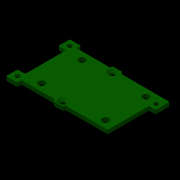
# Autodesk Inventor part: hw_DAA - PCB Sensor
Saved by Autodesk Inventor 2018 (Build 220112000, 112)
## iProperties
Created: 2024-03-13
Part Number: hw_DAA - PCB Sensor
Material: PCB
Document SubType Name: Modeling
Designer: cda1
Density: 4 g/cm^3
Appearance: PCB
Author: cda1
Autodesk Inventor part; units mm, degrees
ref_plane "YZ Plane" through (0, 0, 0) normal (1, 0, 0) x (0, 1, 0)
ref_plane "XZ Plane" through (0, 0, 0) normal (0, 1, 0) x (-1, 0, 0)
ref_plane "XY Plane" through (0, 0, 0) normal (0, 0, 1) x (1, 0, 0)
sketch "Boceto1" plane through (0, 0, 0) normal (0, 0, 1) x (1, 0, 0)
  line L0 (-26, 17) -> (26, 17)
  line L1 (26, 17) -> (26, -17)
  line L2 (26, -17) -> (-26, -17)
  line L3 (-26, -17) -> (-26, 17)
  line L4 (-26, 17) -> (26, -17) construction
  line L5 (26, 17) -> (-26, -17) construction
  point P0 (0, 0)
  dimension "d0" = 52
  dimension "d1" = 34
  constraints: 12 end point, 2 midpoint, 2 parallel, 1 horizontal, 1 perpendicular
  measures "d0" distance of L1.end L2.end
  measures "d1" distance of L0.end L1.end
extrude "Extrusión1" add sketch "Boceto1" against normal blind 1.742
fillet "Empalme1" radius 0.5 4 edges at (26, 17, -0.871) (-26, 17, -0.871) (-26, -17, -0.871) (26, -17, -0.871)
sketch "Boceto2" plane through (0, 0, -1.742) normal (0, 0, -1) x (-1, 0, 0)
  line L0 (-25.5, -17) -> (25.5, -17) projected
  line L1 (-25.5, -17) -> (25.5, -17) projected
  line L2 (22.8, -17) -> (26, -17)
  line L3 (26, -17) -> (26, 13)
  line L4 (26, 13) -> (22.8, 13)
  line L5 (22.8, 13) -> (22.8, -17)
  line L6 (26, 16.5) -> (26, -16.5) projected
  point P0 (0, 0)
  dimension "d5" = 3.2
  dimension "d6" = 30
  constraints: 8 end point, 2 parallel, 2 point on line, 1 horizontal, 1 perpendicular
  measures "d5" distance of L4.end L3.end
  measures "d6" distance of L3.end L2.end
extrude "Extrusión2" cut sketch "Boceto2" against normal through all
sketch "Boceto3" plane through (0, 0, -1.742) normal (0, 0, -1) x (-1, 0, 0)
  line L0 (22.8, 13) -> (26, 13) construction
  line L1 (26, 13) -> (26, 16.5) construction
  arc A0 (26, 16.5) -> (25.5, 17) centre (25.5, 16.5) ccw construction
  line L2 (25.5, 17) -> (-25.5, 17) construction
  arc A1 (-25.5, 17) -> (-26, 16.5) centre (-25.5, 16.5) ccw projected
  line L3 (-26, 16.5) -> (-26, -16.5) projected
  arc A2 (-26, -16.5) -> (-25.5, -17) centre (-25.5, -16.5) ccw projected
  line L4 (-25.5, -17) -> (22.8, -17) construction
  line L5 (22.8, -17) -> (22.8, 13) construction
  line L6 (25.5, 17) -> (-25.5, 17) projected
  line L7 (-25.5, 17) -> (-33.8, 17)
  line L8 (-33.8, 17) -> (-33.8, -17)
  arc A3 (-26, -16.5) -> (-25.5, -17) centre (-25.5, -16.5) ccw projected
  line L9 (-25.5, -17) -> (-33.8, -17)
  point P0 (0, 0)
  dimension "d10" = 8.3
  constraints: 6 end point, 1 collinear, 1 horizontal, 1 perpendicular
  measures "d10" distance of L2.end L7.end
extrude "Extrusión3" add sketch "Boceto3" against normal up to surface (1.742 mm away)
fillet "Empalme2" radius 3.5 2 edges at (33.8, -17, -0.871) (33.8, 17, -0.871)
fillet "Empalme3" radius 1 1 edges at (-22.8, -17, -0.871)
sketch "Boceto4" plane through (0, 0, -1.742) normal (0, 0, -1) x (-1, 0, 0)
  line L0 (-33.8, 13.5) -> (-33.8, -13.5) projected
  line L1 (-30.3, -17) -> (21.8, -17) projected
  line L2 (25.5, 17) -> (-30.3, 17) projected
  line L3 (26, 13) -> (26, 16.5) projected
  point P0 (0, 0)
  point P1 (-24.195, -13.82)
  point P2 (-30.62, 8.694)
  point P3 (18.5, 13.82)
  dimension "d15" = 9.605
  dimension "d16" = 3.18
  dimension "d17" = 8.306
  dimension "d18" = 3.18
  dimension "d19" = 7.5
  dimension "d20" = 3.18
  measures "d15" distance from line of L0 point (-24.195, -13.82)
  measures "d16" distance from line of L1 point (-24.195, -13.82)
  measures "d17" distance from line of L2 point (-30.62, 8.694)
  measures "d18" distance from line of L0 point (-30.62, 8.694)
  measures "d19" distance from line of L3 point (18.5, 13.82)
  measures "d20" distance from line of L2 point (18.5, 13.82)
hole "Agujero1" [suppressed]
sketch "Boceto11" plane through (0, 0, -1.742) normal (0, 0, -1) x (-1, 0, 0)
  line L0 (25.5, 17) -> (-30.3, 17) projected
  line L1 (16.4, 13.533) -> (16.4, -13.067)
  line L2 (-30.3, -17) -> (21.8, -17) projected
  line L3 (22.8, -16) -> (22.8, 13) projected
  line L4 (-33.8, 13.5) -> (-33.8, -13.5) projected
  line L5 (-32.8, 13.533) -> (16.4, 13.533)
  line L6 (-32.8, 13.533) -> (-32.8, -13.067)
  line L7 (-32.8, -13.067) -> (16.4, -13.067)
  line L8 (6.1, -14.067) -> (11.1, -14.067)
  line L9 (11.1, -14.067) -> (11.1, -13.067)
  line L10 (6.1, -14.067) -> (6.1, -13.067)
  line L11 (14.6, 13.533) -> (14.6, 14.533)
  line L12 (14.6, 14.533) -> (9.6, 14.533)
  line L13 (9.6, 14.533) -> (9.6, 13.533)
  line L14 (-32.8, 11.333) -> (-33.8, 11.333)
  line L15 (-32.8, 6.333) -> (-33.8, 6.333)
  line L16 (-33.8, 6.333) -> (-33.8, 11.333)
  arc A0 (-30.3, 17) -> (-33.8, 13.5) centre (-30.3, 13.5) ccw projected
  arc A1 (-33.8, -13.5) -> (-30.3, -17) centre (-30.3, -13.5) ccw projected
  arc A2 (21.8, -17) -> (22.8, -16) centre (21.8, -16) ccw projected
  line L17 (22.8, 13) -> (26, 13) projected
  line L18 (26, 13) -> (26, 16.5) projected
  arc A3 (26, 16.5) -> (25.5, 17) centre (25.5, 16.5) ccw projected
  point P0 (0, 0)
  dimension "d75" = 6.4
  dimension "d76" = 3.467
  dimension "d77" = 1
  dimension "d78" = 3.933
  dimension "d79" = 2.933
  dimension "d80" = 5
  dimension "d81" = 5.3
  dimension "d82" = 5
  dimension "d83" = 1.8
  dimension "d84" = 1
  dimension "d85" = 5
  dimension "d86" = 2.2
  constraints: 26 end point, 9 perpendicular, 8 point on line, 3 vertical, 1 horizontal
  measures "d75" distance between parallel lines of L3 L1
  measures "d76" distance between parallel lines of L0 L5
  measures "d77" distance between parallel lines of L4 L6
  measures "d78" distance between parallel lines of L2 L7
  measures "d79" distance between parallel lines of L2 L8
  measures "d80" distance of L8.start L8.end
  measures "d81" distance from line of L1 L8.end
  measures "d82" distance of L11.end L12.end
  measures "d83" distance between parallel lines of L1 L11
  measures "d84" distance between parallel lines of L5 L12
  measures "d85" distance between parallel lines of L14 L15
  measures "d86" distance between parallel lines of L5 L14
extrude "Extrusión8" cut sketch "Boceto11" against normal through all contours A3 L18 L17 L3 A2 L2 A1 L4 L15 L6 L7 L10 L8 L9 L1 L5 L11 L12 L13 L14 A0 L0
fillet "Empalme5" radius 0.5 16 edges at (32.8, 13.533, -0.871) (32.8, 11.333, -0.871) (33.8, 11.333, -0.871) (33.8, 6.333, -0.871) (32.8, 6.333, -0.871) (32.8, -13.067, -0.871) (-6.1, -13.067, -0.871) (-6.1, -14.067, -0.871) (-11.1, -14.067, -0.871) (-11.1, -13.067, -0.871) (-16.4, -13.067, -0.871) (-16.4, 13.533, -0.871) (-14.6, 13.533, -0.871) (-14.6, 14.533, -0.871) (-9.6, 14.533, -0.871) (-9.6, 13.533, -0.871)
sketch "Boceto13" plane through (0, 0, -1.742) normal (0, 0, -1) x (-1, 0, 0)
  line L0 (9.1, 13.533) -> (-32.3, 13.533) projected
  line L1 (-32.8, 13.033) -> (-32.8, 11.833) projected
  line L2 (-32.3, -13.067) -> (5.6, -13.067) projected
  line L3 (-32.8, 5.833) -> (-32.8, -12.567) projected
  line L4 (16.4, -12.567) -> (16.4, 13.033) projected
  point P0 (0, 0)
  point P1 (3.9, 9.233)
  point P2 (3.9, -8.767)
  point P3 (-24.5, 9.233)
  point P4 (-24.5, -8.767)
  dimension "d103" = 4.3
  dimension "d105" = 4.3
  dimension "d137" = 12.5
  dimension "d188" = 28.4
  constraints: 2 horizontal alignment, 2 vertical alignment
  measures "d103" distance from line of L0 point (3.9, 9.233)
  measures "d105" distance from line of L2 point (3.9, -8.767)
  measures "d137" distance from line of L4 point (3.9, -8.767)
  measures "d188" distance of point (3.9, 9.233) point (-24.5, 9.233)
hole "Agujero5" at (-3.9, 9.233, -1.742) at (-3.9, -8.767, -1.742) at (24.5, 9.233, -1.742) at (24.5, -8.767, -1.742) direction (0, 0, 1) diameter 3 end through all
sketch "Boceto15" plane through (0, 0, 0) normal (0, 0, 1) x (1, 0, 0)
  line L0 (-16.4, 13.033) -> (-16.4, -12.567) projected
  line L1 (32.3, 13.533) -> (-9.1, 13.533) projected
  line L2 (-5.6, -13.067) -> (32.3, -13.067) projected
  point P0 (0, 0)
  point P1 (7.65, 11.233)
  point P2 (7.65, -10.767)
  dimension "d126" = 24.05
  dimension "d127" = 2.3
  dimension "d128" = 2.3
  constraints: 1 vertical alignment
  measures "d126" distance from line of L0 point (7.65, -10.767)
  measures "d127" distance from line of L1 point (7.65, 11.233)
  measures "d128" distance from line of L2 point (7.65, -10.767)
hole "Agujero7" at (7.65, 11.233, 0) at (7.65, -10.767, 0) direction (0, 0, -1) diameter 2 end through all countersink diameter 4 countersink angle 90
sketch "Boceto16" plane through (0, 0, -1.742) normal (0, 0, -1) x (-1, 0, 0)
  circle A0 centre (-24.5, 9.233) radius 1.5 projected
  circle A1 centre (3.9, 9.233) radius 1.5 projected
  circle A2 centre (3.9, -8.767) radius 1.5 projected
  circle A3 centre (3.9, -8.767) radius 2.65
  circle A4 centre (3.9, 9.233) radius 2.65
  circle A5 centre (-24.5, 9.233) radius 2.65
  circle A6 centre (-24.5, -8.767) radius 1.5 projected
  circle A7 centre (-24.5, -8.767) radius 2.65
  point P0 (0, 0)
  dimension "d138" = 5.3
  dimension "d139" = 5.3
  dimension "d140" = 5.3
  dimension "d183" = 5.3
  constraints: 4 centre point, 4 coincident
  measures "d138" diameter of A3
  measures "d139" diameter of A4
  measures "d140" diameter of A5
  measures "d183" diameter of A7
extrude "Extrusión9" add sketch "Boceto16" along normal blind 0.0001
sketch "Boceto18" plane through (0, 0, -1.742) normal (0, 0, -1) x (-1, 0, 0)
  line L0 (12.1724, -6.0157) -> (12.1724, 6.9843) projected
  line L1 (12.1724, 6.9843) -> (13.1724, 6.9843) construction
  line L2 (13.1724, 6.9843) -> (15.6724, 6.9843) construction
  line L3 (13.1724, -6.0157) -> (12.1724, -6.0157) construction
  line L4 (15.6724, -6.0157) -> (13.1724, -6.0157) construction
  line L5 (12.1724, 6.9843) -> (12.1724, 7.9843)
  line L6 (12.1724, 7.9843) -> (16.4, 7.9843)
  line L7 (12.1724, -6.0157) -> (12.1724, -7.0157)
  line L8 (12.1724, -7.0157) -> (16.4, -7.0157)
  line L9 (16.4, -12.567) -> (16.4, 13.033) projected
  line L10 (16.4, -7.0157) -> (16.4, 7.9843)
  point P0 (0, 0)
  dimension "d145" = 1
  dimension "d146" = 1
  constraints: 10 end point, 2 perpendicular, 2 vertical, 1 collinear, 1 point on line
  measures "d145" distance of L0.end L5.end
  measures "d146" distance of L0.start L7.end
extrude "Extrusión11" cut sketch "Boceto18" against normal up to surface (1.742 mm away)
fillet "Empalme6" radius 0.5 2 edges at (-16.4, 7.9843, -0.871) (-16.4, -7.0157, -0.871)
sketch "Boceto19" plane through (0, 0, 0) normal (0, 0, 1) x (1, 0, 0)
  line L0 (-16.4, 13.533) -> (-14.6, 13.533)
  line L1 (-14.6, 13.533) -> (-14.6, -13.067)
  line L2 (-14.6, -13.067) -> (-16.4, -13.067)
  line L3 (-16.4, -13.067) -> (-16.4, 13.533)
  line L4 (-16.4, 8.4843) -> (-16.4, 13.033) projected
  line L5 (-16.4, 9.333) -> (-11.2, 9.333)
  line L6 (-11.2, 9.333) -> (-11.2, -8.867)
  line L7 (-11.2, -8.867) -> (-16.4, -8.867)
  line L8 (-16.4, -8.867) -> (-16.4, 9.333)
  line L9 (-9.6, 13.533) -> (5.4, 13.533)
  line L10 (5.4, 13.533) -> (5.4, 12.533)
  line L11 (5.4, 12.533) -> (-9.6, 12.533)
  line L12 (-9.6, 12.533) -> (-9.6, 13.533)
  line L13 (9.9, 13.533) -> (32.8, 13.533)
  line L14 (32.8, 13.533) -> (32.8, 12.533)
  line L15 (32.8, 12.533) -> (9.9, 12.533)
  line L16 (9.9, 12.533) -> (9.9, 13.533)
  line L17 (32.8, 6.333) -> (31.8, 6.333)
  line L18 (31.8, 6.333) -> (31.8, -13.067)
  line L19 (31.8, -13.067) -> (32.8, -13.067)
  line L20 (32.8, -13.067) -> (32.8, 6.333)
  line L21 (9.9, -12.067) -> (32.8, -12.067)
  line L22 (32.8, -12.067) -> (32.8, -13.067)
  line L23 (32.8, -13.067) -> (9.9, -13.067)
  line L24 (9.9, -13.067) -> (9.9, -12.067)
  line L25 (5.4, -12.067) -> (-9.6, -12.067)
  line L26 (-9.6, -12.067) -> (-9.6, -14.067)
  line L27 (-9.6, -14.067) -> (5.4, -14.067)
  line L28 (5.4, -14.067) -> (5.4, -12.067)
  line L29 (31.8, 13.533) -> (33.8, 13.533)
  line L30 (33.8, 13.533) -> (33.8, 11.333)
  line L31 (33.8, 11.333) -> (31.8, 11.333)
  line L32 (31.8, 11.333) -> (31.8, 13.533)
  line L33 (33.8, 11.333) -> (33.7, 11.333)
  line L34 (33.7, 11.333) -> (33.7, 5.833)
  line L35 (33.7, 5.833) -> (33.8, 5.833)
  line L36 (33.8, 5.833) -> (33.8, 11.333)
  line L37 (33.8, 5.833) -> (32.8, 5.833)
  line L38 (32.8, 5.833) -> (32.8, 6.333)
  line L39 (32.8, 6.333) -> (33.8, 6.333)
  line L40 (33.8, 6.333) -> (33.8, 5.833)
  line L41 (-14.6, 13.533) -> (-16.4, 13.533)
  line L42 (-16.4, 13.533) -> (-16.4, 14.533)
  line L43 (-16.4, 14.533) -> (-14.6, 14.533)
  line L44 (-14.6, 14.533) -> (-14.6, 13.533)
  line L45 (-14.6, 14.533) -> (-9.1, 14.533)
  line L46 (-9.1, 14.533) -> (-9.1, 14.433)
  line L47 (-9.1, 14.433) -> (-14.6, 14.433)
  line L48 (-14.6, 14.433) -> (-14.6, 14.533)
  line L49 (-9.1, 14.533) -> (-9.6, 14.533)
  line L50 (-9.6, 14.533) -> (-9.6, 13.533)
  line L51 (-9.6, 13.533) -> (-9.1, 13.533)
  line L52 (-9.1, 13.533) -> (-9.1, 14.533)
  line L53 (-9.6, -14.067) -> (-11.1, -14.067)
  line L54 (-11.1, -14.067) -> (-11.1, -13.967)
  line L55 (-11.1, -13.967) -> (-9.6, -13.967)
  line L56 (-9.6, -13.967) -> (-9.6, -14.067)
  point P0 (0, 0)
  point P1 (-15.9, 13.533)
  point P2 (-15.9, -13.067)
  point P3 (-11.2, 0.233)
  point P4 (-16.4, 0.233)
  point P5 (32.3, 13.533)
  point P6 (32.8, 13.033)
  point P7 (32.3, -13.067)
  point P8 (32.8, -12.567)
  point P9 (-6.6, -14.067)
  point P10 (32.8, 13.033)
  point P11 (33.75, 5.833)
  point P12 (-14.1, 14.533)
  point P13 (-11.1, -14.017)
  point P14 (-11.1, -13.567)
  dimension "d150" = 1.8
  dimension "d151" = 18.2
  dimension "d152" = 5.2
  dimension "d153" = 1
  dimension "d154" = 15
  dimension "d155" = 0.5
  dimension "d156" = 1
  dimension "d157" = 22.9
  dimension "d158" = 1
  dimension "d159" = 19.4
  dimension "d160" = 1
  dimension "d161" = 2
  dimension "d162" = 22.9
  dimension "d163" = 15
  dimension "d164" = 4.5
  dimension "d165" = 2.2
  dimension "d166" = 2
  dimension "d167" = 1
  dimension "d168" = 0.1
  dimension "d169" = 0.1
  dimension "d170" = 0.1
  constraints: 112 end point, 28 parallel, 14 horizontal, 14 perpendicular, 11 point on line, 8 midpoint, 2 horizontal alignment, 1 vertical alignment
  measures "d150" distance of L0.start L0.end
  measures "d151" distance between parallel lines of L7 L5
  measures "d152" distance of L5.start L5.end
  measures "d153" distance of L9.end L10.end
  measures "d154" distance between parallel lines of L10 L12
  measures "d155" distance from line of L51.end L12
  measures "d156" distance of L15.end L13.start
  measures "d157" distance of L13.start L13.end
  measures "d158" distance of L18.end L19.end
  measures "d159" distance of L19.end L17.start
  measures "d160" distance of L21.end L22.end
  measures "d161" distance of L26.end L25.end
  measures "d162" distance between parallel lines of L22 L24
  measures "d163" distance of L26.end L27.end
  measures "d164" distance between parallel lines of L28 L24
  measures "d165" distance of L29.end L30.end
  measures "d166" distance between parallel lines of L30 L32
  measures "d167" distance from line of L30 point (32.8, 13.033)
  measures "d168" distance of L34.end L35.end
  measures "d169" distance of L45.end L46.end
  measures "d170" distance of L53.end L54.end
extrude "Extrusión12" cut sketch "Boceto19" against normal through all
sketch "Boceto20" plane through (0, 0, -1.742) normal (0, 0, -1) x (-1, 0, 0)
  line L0 (14.6, -13.067) -> (11.6, -13.067) projected
  line L1 (9.6, -13.967) -> (14.6, -13.967)
  line L2 (14.6, -13.967) -> (14.6, -13.067)
  line L3 (14.6, -13.067) -> (9.6, -13.067)
  line L4 (9.6, -13.067) -> (9.6, -13.967)
  point P0 (0, 0)
  constraints: 8 end point, 2 parallel, 1 horizontal, 1 perpendicular
extrude "Extrusión13" add sketch "Boceto20" against normal up to surface (1.742 mm away)
sketch "Boceto12" plane through (0, 0, -1.742) normal (0, 0, -1) x (-1, 0, 0)
  line L0 (-33.8, 10.833) -> (-33.8, 6.833) construction
  line L1 (9.1, 13.533) -> (-32.3, 13.533) construction
  line L2 (16.4, -12.567) -> (16.4, 13.033) construction
  line L3 (14.1, 14.533) -> (10.1, 14.533) construction
  line L4 (6.6, -14.067) -> (10.6, -14.067) construction
  point P0 (0, 0)
  point P1 (-29.521, 8.811)
  point P2 (12.1, 11.889)
  point P3 (12.1, -11.387)
  dimension "d90" = 4.279
  dimension "d91" = 4.722
  dimension "d92" = 4.3
  dimension "d93" = 2.644
  dimension "d94" = 4.3
  dimension "d95" = 2.68
  measures "d90" distance from line of L0 point (-29.521, 8.811)
  measures "d91" distance from line of L1 point (-29.521, 8.811)
  measures "d92" distance from line of L2 point (12.1, 11.889)
  measures "d93" distance from line of L3 point (12.1, 11.889)
  measures "d94" distance from line of L2 point (12.1, -11.387)
  measures "d95" distance from line of L4 point (12.1, -11.387)
hole "Agujero4" at (29.521, 8.811, -1.742) at (-12.1, 11.889, -1.742) at (-12.1, -11.387, -1.742) direction (0, 0, 1) diameter 2 end through all countersink diameter 4 countersink angle 90
fillet "Empalme7" radius 0.5 24 edges at (31.8, 12.533, -0.871) (31.8, 11.333, -0.871) (33.7, 11.1331, -0.871) (33.7, 6.5329, -0.871) (31.8, 6.333, -0.871) (31.8, -12.067, -0.871) (9.9, -12.067, -0.871) (9.9, -13.067, -0.871) (5.4, -12.067, -0.871) (5.4, -13.067, -0.871) (-9.6, -12.067, -0.871) (-9.6, -13.967, -0.871) (-14.6, -13.967, -0.871) (-14.6, -8.867, -0.871) (-11.2, -8.867, -0.871) (-11.2, 9.333, -0.871) (-14.6, 9.333, -0.871) (-14.4001, 14.433, -0.871) (-9.7999, 14.433, -0.871) (-9.6, 12.533, -0.871) (5.4, 13.533, -0.871) (5.4, 12.533, -0.871) (9.9, 13.533, -0.871) (9.9, 12.533, -0.871)
sketch "Boceto21" plane through (0, 0, -1.742) normal (0, 0, -1) x (-1, 0, 0)
  line L0 (-33.2, 6.333) -> (-32.3, 6.333) construction
  arc A0 (-31.8, 5.833) -> (-32.3, 6.333) centre (-32.3, 5.833) ccw construction
  line L1 (-31.8, 5.833) -> (-31.8, -11.567) construction
  line L2 (-31.3, -12.067) -> (-10.4, -12.067) construction
  line L3 (-32.3, 6.333) -> (-33.2, 6.333) projected
  line L4 (-33.2, 6.333) -> (-30.8, 6.333)
  line L5 (-30.8, 6.333) -> (-30.8, -12.067)
  line L6 (-30.8, -12.067) -> (-33.2, -12.067)
  line L7 (-33.2, -12.067) -> (-33.2, 6.333)
  point P0 (0, 0)
  dimension "d176" = 1
  constraints: 8 end point, 2 parallel, 1 horizontal, 1 perpendicular, 1 point on line
  measures "d176" distance between parallel lines of L1 L5
extrude "Extrusión14" cut sketch "Boceto21" against normal up to surface (1.742 mm away)
fillet "Empalme8" radius 0.5 2 edges at (30.8, 6.333, -0.871) (30.8, -12.067, -0.871)
sketch "Boceto22" plane through (0, 0, -1.742) normal (0, 0, -1) x (-1, 0, 0)
  line L0 (-31.8, 12.033) -> (-31.8, 11.833) projected
  line L1 (-31.8, 11.833) -> (-31.8, 6.333)
  line L2 (-33.2, 6.333) -> (-31.3, 6.333) projected
  line L3 (-31.8, 6.333) -> (-33.7, 6.333)
  line L4 (-33.7, 6.333) -> (-33.7, 11.833)
  line L5 (-33.7, 11.833) -> (-31.8, 11.833)
  point P0 (0, 0)
  point P1 (-33.7, 10.833)
  constraints: 8 end point, 3 point on line, 2 vertical, 1 perpendicular
extrude "Extrusión15" cut sketch "Boceto22" against normal up to surface (1.742 mm away)
fillet "Empalme9" radius 0.5 1 edges at (31.8, 6.333, -0.871)
sketch "Boceto23" plane through (0, 0, 0) normal (0, 0, 1) x (1, 0, 0)
  line L0 (10.4, -12.067) -> (30.3, -12.067) projected
  line L1 (28.8, -12.067) -> (28.8, 6.333)
  line L2 (30.8, -11.567) -> (30.8, 5.833) projected
  arc A0 (31.3, 6.333) -> (30.8, 5.833) centre (31.3, 5.833) ccw projected
  line L3 (28.8, 6.333) -> (31.3, 6.333)
  arc A1 (30.3, -12.067) -> (30.8, -11.567) centre (30.3, -11.567) ccw projected
  point P0 (0, 0)
  dimension "d184" = 2
  constraints: 4 end point, 1 horizontal, 1 point on line, 1 tangent, 1 vertical
  measures "d184" distance between parallel lines of L2 L1
extrude "Extrusión16" cut sketch "Boceto23" against normal up to surface (1.742 mm away)
fillet "Empalme10" radius 0.5 2 edges at (28.8, 6.333, -0.871) (28.8, -12.067, -0.871)
